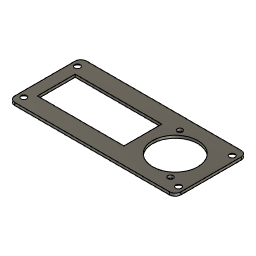
vsps power front plate (Autodesk Fusion 360 design; units mm, degrees)
Autodesk Fusion 360 part; units mm, degrees
sketch "Sketch1" plane through (0, 0, 0) normal (0, 0, 1) x (1, 0, 0)
  line L0 (3, 0) -> (85, 0)
  line L1 (88, 3) -> (88, 35)
  line L2 (85, 38) -> (3, 38)
  line L3 (0, 35) -> (0, 3)
  arc A0 (0, 3) -> (3, 0) centre (3, 3) ccw
  arc A1 (3, 38) -> (0, 35) centre (3, 35) ccw
  arc A2 (88, 35) -> (85, 38) centre (85, 35) ccw
  arc A3 (85, 0) -> (88, 3) centre (85, 3) ccw
  circle A4 centre (3, 33.2) radius 1.5
  circle A5 centre (3, 4.8) radius 1.5
  circle A6 centre (85, 4.8) radius 1.5
  circle A7 centre (85, 33.2) radius 1.5
  line L4 (6, 29) -> (51.85, 29)
  line L5 (51.85, 29) -> (51.85, 9)
  line L6 (51.85, 9) -> (6, 9)
  line L7 (6, 9) -> (6, 29)
  circle A8 centre (69, 19.0205) radius 12
  circle A9 centre (78.5, 7.0205) radius 1.4
  circle A10 centre (59.5, 31.0205) radius 1.4
  line L8 (59.5, 31.0205) -> (78.5, 7.0205) construction
  line L9 (59, 34.5205) -> (79, 34.5205) construction
  line L10 (82, 31.5205) -> (82, 6.5205) construction
  line L11 (79, 3.5205) -> (59, 3.5205) construction
  line L12 (56, 6.5205) -> (56, 31.5205) construction
  line L13 (56, 34.5205) -> (82, 3.5205) construction
  arc A11 (56, 6.5205) -> (59, 3.5205) centre (59, 6.5205) ccw construction
  arc A12 (82, 31.5205) -> (79, 34.5205) centre (79, 31.5205) ccw construction
  arc A13 (59, 34.5205) -> (56, 31.5205) centre (59, 31.5205) ccw construction
  arc A14 (79, 3.5205) -> (82, 6.5205) centre (79, 6.5205) ccw construction
  line L14 (3, 33.2) -> (85, 33.2) construction
  line L15 (85, 33.2) -> (85, 4.8) construction
  line L16 (85, 4.8) -> (3, 4.8) construction
  line L17 (3, 4.8) -> (3, 33.2) construction
  point P0 (88, 0)
  point P1 (0, 38)
  point P2 (82, 34.5205)
  point P3 (56, 3.5205)
  point P4 (3, 19)
  point P5 (0, 19)
  point P6 (44, 38)
  point P7 (44, 33.2)
  dimension "d1" = 88
  dimension "d2" = 38
  dimension "d3" = 3
  dimension "d5" = 3
  dimension "d8" = 45.85
  dimension "d9" = 20
  dimension "d10" = 9
  dimension "d11" = 6
  dimension "d12" = 24
  dimension "d14" = 2.8
  dimension "d17" = 26
  dimension "d18" = 31
  dimension "d19" = 3
  dimension "d20" = 6
  dimension "d24" = 24
  dimension "d25" = 19
  dimension "d27" = 82
  dimension "d28" = 28.4
  constraint horizontal L0
  constraint vertical L1
  constraint horizontal L2
  constraint vertical L3
  constraint coincident origin L0
  constraint coincident origin L3
  constraint tangent L0 A0
  constraint tangent L3 A0
  constraint coincident P1 L2
  constraint coincident P1 L3
  constraint tangent L2 A1
  constraint tangent L3 A1
  constraint equal A0 A1
  constraint tangent L1 A2
  constraint tangent L2 A2
  constraint equal A0 A2
  constraint coincident P0 L0
  constraint coincident P0 L1
  constraint tangent L0 A3
  constraint tangent L1 A3
  constraint equal A0 A3
  constraint horizontal L4
  constraint vertical L5
  constraint horizontal L6
  constraint vertical L7
  constraint coincident A10.centre L8.start
  constraint coincident A9.centre L8.end
  constraint coincident A8.centre L8
  constraint horizontal L9
  constraint vertical L10
  constraint horizontal L11
  constraint vertical L12
  constraint coincident A8.centre L13
  constraint coincident P3 L11
  constraint coincident P3 L12
  constraint tangent L11 A11
  constraint tangent L12 A11
  constraint coincident P2 L9
  constraint coincident P2 L10
  constraint tangent L9 A12
  constraint tangent L10 A12
  constraint equal A11 A12
  constraint coincident L13.start L12
  constraint coincident L13.start L9
  constraint tangent L12 A13
  constraint tangent L9 A13
  constraint equal A11 A13
  constraint coincident L13.end L10
  constraint coincident L13.end L11
  constraint tangent L10 A14
  constraint tangent L11 A14
  constraint equal A11 A14
  constraint midpoint A8.centre L8
  constraint midpoint A8.centre L13
  constraint equal A9 A10
  constraint equal A4 A5
  constraint equal A5 A6
  constraint equal A6 A7
  constraint horizontal L14
  constraint vertical L15
  constraint horizontal L16
  constraint vertical L17
  constraint coincident A6.centre L15.end
  constraint coincident A4.centre L14.start
  constraint coincident A5.centre L16.end
  constraint coincident L17 P4
  constraint midpoint L17 P4
  constraint coincident L3 P5
  constraint midpoint L3 P5
  constraint horizontal P4 P5
  constraint coincident L2 P6
  constraint coincident L14 P7
  constraint midpoint L2 P6
  constraint midpoint L14 P7
  constraint vertical P6 P7
  constraint coincident A7.centre L14.end
  measures "d1" distance of origin P0
  measures "d2" distance of origin P1
  measures "d3" radius of A0
  measures "d5" diameter of A5
  measures "d8" distance of L4.start L4.end
  measures "d9" distance of L4.start L6.end
  measures "d10" distance of L2 L4
  measures "d11" distance of L3 L7
  measures "d12" diameter of A8
  measures "d14" diameter of A10
  measures "d17" distance of L13.start P2
  measures "d18" distance of L13.start P3
  measures "d19" radius of A11
  measures "d20" distance of L1 L10
  measures "d24" vertical distance of A9.centre A10.centre
  measures "d25" horizontal distance of A9.centre A10.centre
  measures "d27" distance of A4.centre A7.centre
  measures "d28" distance of A4.centre A5.centre
extrude "Extrude1" add sketch "Sketch1" along normal blind 1.4
chamfer "Chamfer2" distance 1.4 angle 45 4 edges at (83.6015, 5.3424, 0) (83.6015, 33.7424, 0) (1.6015, 5.3424, 0) (1.6015, 33.7424, 0)
equation "d10 = ( 38 mm - 20 mm ) / 2"
